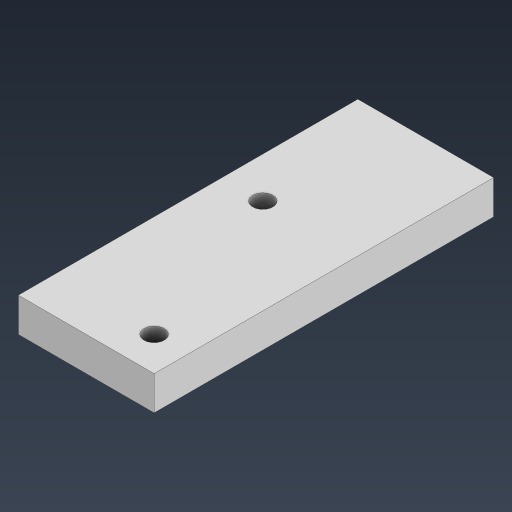
# Autodesk Inventor part: szczeka
Saved by Autodesk Inventor 2024 (Build 280153000, 153)
## iProperties
Created: 2023-12-20
Part Number: szczeka
Material: Generic
Document SubType Name: Modeling
Designer: Piter
Density: 1 g/cm^3
Appearance: Default
Author: Piter
Autodesk Inventor part; units mm, degrees
ref_plane "YZ Plane" through (0, 0, 0) normal (1, 0, 0) x (0, 1, 0)
ref_plane "XZ Plane" through (0, 0, 0) normal (0, 1, 0) x (-1, 0, 0)
ref_plane "XY Plane" through (0, 0, 0) normal (0, 0, 1) x (1, 0, 0)
sketch "Sketch1" plane through (0, 0, 0) normal (0, 1, 0) x (-1, 0, 0)
  line L0 (0, 0) -> (20, 0)
  line L1 (20, 0) -> (20, -50)
  line L2 (20, -50) -> (0, -50)
  line L3 (0, -50) -> (0, 0)
  circle A0 centre (14, -30) radius 1.5
  line L4 (10, 0) -> (10, -50)
  line L5 (0, 0) -> (10, 0)
  circle A1 centre (5, -5) radius 1.5
  line L6 (5, -5) -> (20, -5)
  line L7 (5, -5) -> (5, -50)
  dimension "d0" = 20
  dimension "d1" = 50
  dimension "d3" = 3
  dimension "d4" = 3
  dimension "d5" = 5
  dimension "d6" = 5
  dimension "d7" = 25
  dimension "d9" = 9
  constraints: 16 end point, 3 perpendicular, 2 centre point, 2 horizontal, 2 midpoint, 2 parallel, 2 point on line
  measures "d0" distance of L1.end L2.end
  measures "d1" distance of L0.end L1.end
  measures "d3" diameter of A0
  measures "d4" diameter of A1
  measures "d5" distance from line of L4 L6.start
  measures "d6" distance from line of L0 L6.start
  measures "d7" distance from line of A0.centre L6
  measures "d9" distance from line of L7 A0.centre
extrude "Extrusion1" add sketch "Sketch1" along normal blind 5 contours L0 L4 L6 A1 L7 L2 L3 | L0 L1 L6 L4 | L6 L1 L2 L4 | L4 L2 L7 A1 L6
body "Solid1"
